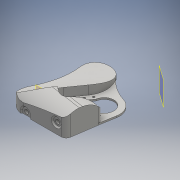
# Autodesk Inventor part: Arm - right shoulder
Saved by Autodesk Inventor 2016 (Build 200138000, 138)
## iProperties
Created: 2016-04-08
Part Number: Arm - right shoulder
Material: Generic
Document SubType Name: Modeling
Designer: alist
Density: 1 g/cm^3
Appearance: Default
Author: alist
Autodesk Inventor part; units mm, degrees
ref_plane "YZ Plane" through (0, 0, 0) normal (1, 0, 0) x (0, 1, 0)
ref_plane "XZ Plane" through (0, 0, 0) normal (0, 1, 0) x (-1, 0, 0)
ref_plane "XY Plane" through (0, 0, 0) normal (0, 0, 1) x (1, 0, 0)
sketch "Sketch1" plane through (0, 0, 0) normal (0, 0, 1) x (1, 0, 0)
  arc A0 (-14.2808, 17.2713) -> (4.3506, -10) centre (4.3506, 10) ccw
  line L0 (4.3506, -10) -> (48.9241, -10)
  arc A1 (48.9241, -10) -> (54.8624, -4.8582) centre (48.9241, -4) ccw
  line L1 (54.8624, -4.8582) -> (58.9912, 23.7095)
  arc A2 (62.1078, 42.0614) -> (58.9912, 23.7095) centre (851.262, -101.3974) ccw
  arc A3 (62.1078, 42.0614) -> (49.584, 62.6445) centre (44.263, 45.3054) ccw
  arc A4 (23.3569, 80.1473) -> (49.584, 62.6445) centre (65.7197, 115.2244) ccw
  arc A5 (23.3569, 80.1473) -> (-6.689, 68.0289) centre (10.263, 69.3054) ccw
  arc A6 (-14.2808, 17.2713) -> (-6.689, 68.0289) centre (-122.075, 59.3405) ccw
  circle A7 centre (44.263, 45.3054) radius 11.15 projected
  line L2 (4.3506, -5) -> (4.3506, -16.4137) construction
  line L3 (48.9241, -5) -> (48.9241, -18.2339) construction
  line L4 (44.263, 45.3054) -> (44.263, 121.9017) construction
  line L5 (44.263, 45.3054) -> (10.263, 69.3054) construction
  point P0 (26.3348, -5)
  point P1 (37.9241, -5)
  dimension "d0" = 34
  dimension "d1" = 24
  dimension "d2" = 17
  dimension "d3" = 18.1372
  dimension "d4" = 6
  dimension "d5" = 20
  dimension "d6" = 115.7126
  dimension "d7" = 55
  dimension "d8" = 5
  dimension "d65" = 54.782
  constraints: 14 point on circle, 12 end point, 8 tangent, 7 centre point, 3 vertical, 2 point on line, 1 coincident, 1 horizontal, 4 other
  measures "d0" horizontal distance of A3.centre L5.end
  measures "d1" vertical distance of A3.centre L5.end
  measures "d2" radius of A5
  measures "d3" radius of A3
  measures "d4" radius of A1
  measures "d5" radius of A0
  measures "d6" radius of A6
  measures "d7" radius of A4
  measures "d8" distance from line of L0 point (26.335, -5)
  measures "d65" angle of L5 L4
extrude "Extrusion1" add sketch "Sketch1" along normal blind 4.1125
sketch "Sketch2" plane through (0, 0, 4.1125) normal (0, 0, 1) x (1, 0, 0)
  line L0 (12.6677, 29.6627) -> (35.4339, 61.9148) construction
  arc A0 (12.6677, 29.6627) -> (14.7201, 17.7589) centre (19.6458, 24.737) ccw projected
  line L1 (28.2001, 8.2436) -> (14.7201, 17.7589) projected
  arc A1 (28.2001, 8.2436) -> (40.1039, 10.296) centre (33.1258, 15.2217) ccw projected
  line L2 (56.8231, 33.9816) -> (40.1039, 10.296) construction
  circle A2 centre (44.263, 45.3054) radius 11.15 projected
  arc A3 (-14.2808, 17.2713) -> (4.3506, -10) centre (4.3506, 10) ccw projected
  line L3 (4.3506, -10) -> (48.9241, -10) projected
  arc A4 (48.9241, -10) -> (54.8624, -4.8582) centre (48.9241, -4) ccw projected
  line L4 (54.8624, -4.8582) -> (58.9912, 23.7095) projected
  arc A5 (62.1078, 42.0614) -> (58.9912, 23.7095) centre (851.262, -101.3974) ccw projected
  arc A6 (62.1078, 42.0614) -> (49.584, 62.6445) centre (44.263, 45.3054) ccw projected
  arc A7 (23.3569, 80.1473) -> (49.584, 62.6445) centre (65.7197, 115.2244) ccw projected
  arc A8 (23.3569, 80.1473) -> (-6.689, 68.0289) centre (10.263, 69.3054) ccw projected
  arc A9 (-14.2808, 17.2713) -> (-6.689, 68.0289) centre (-122.075, 59.3405) ccw projected
  arc A10 (23.3569, 80.1473) -> (49.584, 62.6445) centre (65.7197, 115.2244) ccw projected
  line L5 (24.6467, 46.6329) -> (12.6677, 29.6627)
  line L6 (54.8624, -4.8582) -> (58.9912, 23.7095) projected
  arc A11 (58.9912, 23.7095) -> (51.6396, 26.6382) centre (54.9639, 24.2916) ccw
  line L7 (51.6396, 26.6382) -> (40.1039, 10.296)
  arc A12 (23.3569, 80.1473) -> (-6.689, 68.0289) centre (10.263, 69.3054) ccw projected
  arc A13 (24.6467, 46.6329) -> (23.3569, 80.1473) centre (2.1013, 62.5473) ccw
  point P0 (0, 0)
  constraints: 5 tangent, 4 end point, 4 point on circle, 2 centre point, 2 collinear, 2 point on line
extrude "Extrusion2" cut sketch "Sketch2" against normal blind 2.1125 contours L5 A13 A7 A6 A5 A11 L7 A1 L1 A0
sketch "Sketch3" plane through (0, 0, 4.1125) normal (0, 0, 1) x (1, 0, 0)
  arc A0 (58.9912, 23.7095) -> (51.6396, 26.6382) centre (54.9639, 24.2916) ccw projected
  line L0 (51.6396, 26.6382) -> (40.1039, 10.296) projected
  arc A1 (28.2001, 8.2436) -> (40.1039, 10.296) centre (33.1258, 15.2217) ccw projected
  line L1 (28.2001, 8.2436) -> (14.7201, 17.7589) projected
  arc A2 (12.6677, 29.6627) -> (14.7201, 17.7589) centre (19.6458, 24.737) ccw projected
  line L2 (12.6677, 29.6627) -> (24.6467, 46.6329) projected
  arc A3 (24.6467, 46.6329) -> (23.3569, 80.1473) centre (2.1013, 62.5473) ccw construction
  arc A4 (23.3569, 80.1473) -> (-6.689, 68.0289) centre (10.263, 69.3054) ccw projected
  arc A5 (-14.2808, 17.2713) -> (-6.689, 68.0289) centre (-122.075, 59.3405) ccw construction
  arc A6 (-14.2808, 17.2713) -> (4.3506, -10) centre (4.3506, 10) ccw projected
  line L3 (4.3506, -10) -> (48.9241, -10) projected
  arc A7 (48.9241, -10) -> (54.8624, -4.8582) centre (48.9241, -4) ccw projected
  line L4 (54.8624, -4.8582) -> (58.9912, 23.7095) projected
  arc A8 (6.5427, 23.5311) -> (-14.2808, 17.2713) centre (-1.4192, 12.2518) ccw
  line L5 (28.2001, 8.2436) -> (14.7201, 17.7589) projected
  line L6 (12.8052, 19.1105) -> (6.5427, 23.5311)
  arc A9 (28.082, 71.8513) -> (-6.4058, 62.512) centre (10.263, 69.3054) ccw
  arc A10 (-14.2808, 17.2713) -> (-6.689, 68.0289) centre (-122.075, 59.3405) ccw projected
  arc A11 (-14.2808, 17.2713) -> (-6.4058, 62.512) centre (-122.075, 59.3405) ccw
  arc A12 (-6.4058, 62.512) -> (28.082, 71.8513) centre (10.263, 69.3054) ccw
  arc A13 (24.6467, 46.6329) -> (23.3569, 80.1473) centre (2.1013, 62.5473) ccw projected
  arc A14 (24.6467, 46.6329) -> (28.082, 71.8513) centre (2.1013, 62.5473) ccw
  point P0 (0, 0)
  dimension "d15" = 36
  constraints: 14 point on circle, 5 centre point, 3 coincident, 2 end point, 2 tangent, 1 collinear, 1 point on line
  measures "d15" diameter of A9
extrude "Extrusion3" add sketch "Sketch3" along normal blind 22 contours L4 A7 L3 A6 A10 A12 A13 L2 A2 L1 A1 L0 A0 | A10 A4 A13 A12
ref_plane "Work Plane1" through (78.9482, 80.1368, 26.1125) normal (0.5766832, 0.8169679, 0) x (0.8169679, -0.5766832, 0)
sketch "Sketch4" plane through (78.9482, 80.1368, 26.1125) normal (0.5766832, 0.8169679, 0) x (0.8169679, -0.5766832, 0)
  line L0 (0, 0) -> (-16.5, 0) projected
  line L1 (-66.8673, 22) -> (-45.4224, 22) projected
  arc A0 (-8.25, 0) -> (-56.1448, 22) centre (-56.7698, -42.495) ccw
  circle A1 centre (-56.7698, -42.495) radius 64.498
  point P0 (-18.2846, 26.1125)
  point P1 (-17.6719, 0)
  point P2 (-62.9804, 22)
  constraints: 2 centre point, 2 midpoint, 2 point on circle, 1 coincident, 1 concentric
extrude "Extrusion4" cut sketch "Sketch4" against normal blind 128.25
sketch "Sketch5" plane through (58.9912, 23.7095, 2) normal (0.9897169, -0.14304, 0) x (0, 0, -1)
  line L0 (0, 4.0691) -> (-24.1125, 4.0691) projected
  line L1 (2, -41.1787) -> (-23.3114, -41.1787) projected
  arc A0 (-12.2178, 4.0691) -> (-10.6557, -41.1787) centre (2.343, -18.0791) ccw
  arc A1 (-12.2178, 4.0691) -> (-10.6557, -41.1787) centre (-44.9361, -19.7113) ccw
  point P0 (2, -31.9038)
  point P1 (-24.1125, -19.7113)
  constraints: 5 point on circle, 2 centre point, 1 midpoint, 1 point on line
extrude "Extrusion5" cut sketch "Sketch5" against normal blind 128.25
sketch "Sketch6" plane through (4.3506, -10, 0) normal (0, -1, 0) x (1, 0, 0)
  line L0 (44.5735, 0) -> (44.5735, 12.1598) construction
  arc A0 (44.5735, 12.1598) -> (33.5735, 12.1598) centre (39.0735, 12.1598) ccw construction
  line L1 (33.5735, 12.1598) -> (33.5735, 0) construction
  line L2 (21.9842, 0) -> (21.9842, 7.9691) construction
  arc A1 (21.9842, 7.9691) -> (15.481, 13.3768) centre (16.4842, 7.9691) ccw construction
  line L3 (15.481, 13.3768) -> (4.4968, 11.339) construction
  arc A2 (4.4968, 11.339) -> (0, 5.9313) centre (5.5, 5.9313) ccw construction
  line L4 (0, 5.9313) -> (0, 0) construction
  line L5 (32.5735, 0) -> (32.5735, 12.1598)
  arc A3 (45.5735, 12.1598) -> (32.5735, 12.1598) centre (39.0735, 12.1598) ccw
  line L6 (45.5735, 12.1598) -> (45.5735, 0)
  line L7 (-1, 0) -> (-1, 5.9313)
  arc A4 (4.3143, 12.3222) -> (-1, 5.9313) centre (5.5, 5.9313) ccw
  line L8 (4.3143, 12.3222) -> (15.2986, 14.36)
  arc A5 (22.9842, 7.9691) -> (15.2986, 14.36) centre (16.4842, 7.9691) ccw
  line L9 (22.9842, 7.9691) -> (22.9842, 0)
  line L10 (32.5735, 0) -> (45.5735, 0)
  line L11 (22.9842, 0) -> (-1, 0)
  point P0 (-4.3506, 0)
  dimension "d22" = 1
  dimension "d23" = 1
  constraints: 14 end point, 6 point on circle, 3 centre point, 2 perpendicular, 6 other
  measures "d22" distance between parallel lines of L1 L5
  measures "d23" radial gap between concentric circles of A1 A5
extrude "Extrusion6" add sketch "Sketch6" against normal blind 34.5 separate body
sketch "Sketch7" plane through (0, 0, 0) normal (0, 0, -1) x (-1, 0, 0)
  line L0 (-26.3348, -5) -> (-4.3506, -5) construction
  line L1 (-19.8316, 0) -> (-8.8474, 0) construction
  line L2 (-70.1929, 0) -> (0, 0)
  line L3 (-70.1929, -5) -> (0, -5)
  line L4 (-70.1929, -5) -> (-70.1929, 0)
  line L5 (0, -5) -> (0, 0)
  constraints: 8 end point, 2 horizontal, 2 point on line, 1 perpendicular, 1 vertical
extrude "Extrusion7" cut sketch "Sketch7" against normal blind 34.5 keep common part bodies 2
combine bodies "Combine1" operation type subtract main body 1 bodies to subtract 2
chamfer "Chamfer1" distance 2 angle 45 4 edges at (43.4241, 0, 0) (43.4241, -5, 0) (15.3427, 0, 0) (15.3427, -5, 0)
sketch "Sketch8" plane through (4.3506, -10, 0) normal (0, -1, 0) x (1, 0, 0)
  circle A0 centre (39.051, 12.0643) radius 2.15 projected
  circle A1 centre (2.6827, 4) radius 2.15 projected
  point P0 (-4.3506, 0)
hole "Hole1" at (43.4016, -10, 12.0643) at (7.0333, -10, 4) direction (0, 1, 0) diameter 4.7 depth 40 tip angle 118 bodies 1
sketch "Sketch9" plane through (4.3506, -10, 0) normal (0, -1, 0) x (1, 0, 0)
  circle A0 centre (2.6827, 4) radius 2.35 projected
  circle A1 centre (39.051, 12.0643) radius 2.35 projected
  line L0 (2.6827, 4) -> (2.6827, -7.8438) construction
  line L1 (-1.8173, 4) -> (-1.8173, -7.8438)
  line L2 (7.1827, -7.8438) -> (7.1827, 4)
  arc A2 (7.1827, 4) -> (-1.8173, 4) centre (2.6827, 4) ccw
  arc A3 (-1.8173, -7.8438) -> (7.1827, -7.8438) centre (2.6827, -7.8438) ccw
  circle A4 centre (39.051, 12.0643) radius 2.35 projected
  circle A5 centre (39.051, 12.0643) radius 4.5
  point P0 (-4.3506, 0)
  point P1 (2.6827, -1.9219)
  dimension "d41" = 9
  dimension "d42" = 9
  constraints: 8 end point, 4 point on circle, 4 tangent, 3 centre point, 1 coincident, 1 midpoint, 1 parallel, 1 vertical
  measures "d41" diameter of A3
  measures "d42" diameter of A5
extrude "Extrusion8" cut sketch "Sketch9" against normal blind 1.5 bodies 1
chamfer "Chamfer3" distance 1.417 angle 45 5 edges at (11.5333, -10, 2) (9.0554, -10, 8.0201) (2.9694, -9.9522, 5.9324) (2.5333, -9.9173, 2) (38.9016, -10, 12.0643)
ref_plane "Work Plane2" through (12.9503, 7, 0) normal (0, -1, 0) x (1, 0, 0)
sketch "Sketch10" plane through (12.9503, 7, 0) normal (0, -1, 0) x (1, 0, 0)
  circle A0 centre (30.4513, 12.0643) radius 2.35 projected
  line L0 (26.8013, 14.1717) -> (30.4513, 16.279)
  line L1 (30.4513, 16.279) -> (34.1013, 14.1717)
  line L2 (34.1013, 14.1717) -> (34.1013, 9.957)
  line L3 (34.1013, 9.957) -> (30.4513, 7.8497)
  line L4 (30.4513, 7.8497) -> (26.8013, 9.957)
  line L5 (26.8013, 9.957) -> (26.8013, 14.1717)
  arc A1 (-4.6831, 2) -> (-7.1509, 2) centre (-5.917, 4) ccw projected
  line L6 (-3.8097, 0.35) -> (-8.0243, 0.35)
  line L7 (-8.0243, 0.35) -> (-10.1317, 4)
  line L8 (-10.1317, 4) -> (-8.0243, 7.65)
  line L9 (-8.0243, 7.65) -> (-3.8097, 7.65)
  line L10 (-3.8097, 7.65) -> (-1.7023, 4)
  line L11 (-1.7023, 4) -> (-3.8097, 0.35)
  line L12 (46.376, -6.7597) -> (-18.4754, -6.7597)
  line L13 (-1.7023, 4) -> (-1.7023, -6.7597)
  line L14 (-10.1317, 4) -> (-10.1317, -6.7597)
  line L15 (-10.1317, 4) -> (-1.7023, 4) construction
  line L16 (34.1013, 12.0643) -> (26.8013, 12.0643) construction
  line L17 (34.1013, 9.957) -> (34.1013, -6.7597)
  line L18 (26.8013, 9.957) -> (26.8013, -6.7597)
  point P0 (-12.9503, 0)
  dimension "d49" = 7.3
  dimension "d50" = 7.3
  constraints: 38 end point, 4 perpendicular, 4 point on line, 2 coincident, 2 midpoint, 2 parallel, 1 horizontal, 26 other
  measures "d49" distance between parallel lines of L8 L11
  measures "d50" distance between parallel lines of L1 L4
extrude "Extrusion9" cut sketch "Sketch10" along normal blind 3.2 and the other way blind 1 contours A0 | L0 L1 L2 L3 L4 L5 | L4 L3 L17 L12 L18 | L11 L13 L12 L14 L7 L6 | L6 L7 L8 L9 L10 L11 bodies 1
sketch "Sketch12" plane through (0, 0, 0) normal (0, 0, -1) x (-1, 0, 0)
  line L0 (-33.0116, 47.1399) -> (-18.0119, 25.8904)
  arc A0 (-18.4925, 23.1031) -> (-18.0119, 25.8904) centre (-19.6458, 24.737) ccw
  line L1 (-18.4925, 23.1031) -> (-31.9724, 13.5878)
  arc A1 (-34.7597, 14.0684) -> (-31.9724, 13.5878) centre (-33.1258, 15.2217) ccw
  line L2 (-34.7597, 14.0684) -> (-49.7594, 35.3179)
  arc A2 (-33.0116, 47.1399) -> (-49.7594, 35.3179) centre (-44.263, 45.3054) ccw
  point P0 (0, 0)
  dimension "d64" = 11.4
  constraints: 6 end point, 6 point on circle, 3 centre point, 2 tangent, 1 parallel, 6 other
  measures "d64" radius of A2
extrude "Extrusion10" cut sketch "Sketch12" against normal blind 2 bodies 1
sketch "Sketch13" plane through (0, 0, 0) normal (0, 0, -1) x (-1, 0, 0)
  circle A0 centre (-51.5436, 32.2099) radius 1.15 projected
  circle A1 centre (-46.9301, 25.6741) radius 1.15 projected
  circle A2 centre (-42.3167, 19.1384) radius 1.15 projected
  circle A3 centre (-37.7032, 12.6026) radius 1.15 projected
  circle A4 centre (-30.0381, 11.2811) radius 1.15 projected
  circle A5 centre (-16.9666, 20.508) radius 1.15 projected
  circle A6 centre (-15.6451, 28.1731) radius 1.15 projected
  circle A7 centre (-20.2585, 34.7088) radius 1.15 projected
  circle A8 centre (-24.872, 41.2446) radius 1.15 projected
  circle A9 centre (-29.4855, 47.7803) radius 1.15 projected
  point P0 (0, 0)
hole "Hole2" at (51.5436, 32.2099, 0) at (46.9301, 25.6741, 0) at (42.3167, 19.1384, 0) at (37.7032, 12.6026, 0) at (30.0381, 11.2811, 0) at (16.9666, 20.508, 0) at (15.6451, 28.1731, 0) at (20.2585, 34.7088, 0) at (24.872, 41.2446, 0) at (29.4855, 47.7803, 0) direction (0, 0, 1) diameter 2.5 end through all bodies 1
body "Solid1"
